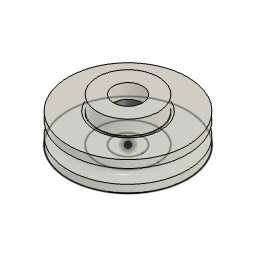
FilamentRoller v3 (Autodesk Fusion 360 design; units mm, degrees)
Autodesk Fusion 360 part; units mm, degrees
sketch "Main" plane through (0, 0, 0) normal (0, 0, 1) x (1, 0, 0)
  circle A0 centre (0, 0) radius 3.125
  circle A1 centre (0, 0) radius 6.125
  circle A2 centre (0, 0) radius 1.5
  dimension "d1" = 6.25
  dimension "d3" = 3
  dimension "d12" = 3
  constraint coincident A0.centre A1.centre
  measures "d1" diameter of A0
  measures "d12" diameter of A2
extrude "Extrude1" add sketch "Main" along normal blind 3 contours A1 makes body 1
sketch "Sketch2" plane through (0, 0, 0) normal (1, 0, 0) x (0, 1, 0)
  line L0 (6.125, 3) -> (-6.125, 3)
  line L1 (6.125, 0) -> (-6.125, 0)
  line L2 (6.125, 3) -> (6.125, 0)
  line L3 (6.125, 1.5) -> (5.125, 1.5) construction
  spline S0 degree 5 poles (6.125, 3) (6.125, 2.8466) (6.1777, 2.5757) (6.4146, 2.2769) (6.9886, 2.0773) (7.8292, 2.0694) (8.4441, 2.1927) (8.5459, 2.3381) (8.0488, 2.4223) (7.1302, 2.4004) (6.0916, 2.2496) (5.4387, 2.0191) (5.1775, 1.7838) (5.1226, 1.5992) (5.125, 1.5) knots 0 0 0 0 0 0 0.1 0.2 0.3 0.4 0.5 0.6 0.7 0.8 0.9 1 1 1 1 1 1
  line L4 (6.125, 3.25) -> (6.125, 2.75)
  line L5 (5.122, 1.6259) -> (5.128, 1.3741)
  spline S1 degree 5 poles (6.125, 0) (6.125, 0.1534) (6.1777, 0.4243) (6.4146, 0.7231) (6.9886, 0.9227) (7.8292, 0.9306) (8.4441, 0.8073) (8.5459, 0.6619) (8.0488, 0.5777) (7.1302, 0.5996) (6.0916, 0.7504) (5.4387, 0.9809) (5.1775, 1.2162) (5.1226, 1.4008) (5.125, 1.5) knots 0 0 0 0 0 0 0.1 0.2 0.3 0.4 0.5 0.6 0.7 0.8 0.9 1 1 1 1 1 1
  line L6 (6.125, -0.25) -> (6.125, 0.25)
  line L7 (5.122, 1.3741) -> (5.128, 1.6259)
  point P0 (8.4316, 2.2871)
  point P1 (8.4316, 0.7129)
  dimension "d8" = 1
  constraint coincident L0.start L2.start
  constraint coincident L1.start L2.end
  constraint midpoint L2 L3.start
  constraint perpendicular L2 L3
  constraint midpoint L0.start L4
  constraint coincident L2 L4.end
  constraint midpoint L3.end L5
  constraint symmetric S0.end L3 S1.end
  constraint symmetric L3 L0.start L1.start
  constraint symmetric L3 P0 P1
  constraint symmetric L3 L4.start L6.start
  constraint symmetric L3 L4.end L6.end
  constraint symmetric L3 L5.start L7.start
  constraint symmetric L3 L5.end L7.end
  measures "d8" distance of L3.start L3.end
revolve "Revolve1" cut sketch "Sketch2" angle 360 about axis through (0, 0, 0) along (0, 0, -1) contours L2 S0 S1 bodies 1
fillet "Fillet1" radius 0.25 2 edges at (-2.9135, 1.13, 3) (-2.9135, 1.13, 0) on bodies 1
extrude "Extrude2" add sketch "Main" along normal blind 3 separate body contours A0 makes body 2
sketch "Sketch3" plane through (0, 0, 3) normal (0, 0, 1) x (-1, 0, 0)
  circle A0 centre (0, 0) radius 1.5
  circle A1 centre (0, 0) radius 3.125
extrude "Extrude3" add sketch "Sketch3" along normal blind 1.5 separate body makes body 3
copy_body "CopyPasteBodies1" bodies 3 makes body 4
move_body "Move1" bodies 4 to x (1, 0, 0) y (0, 1, 0) z (0, 0, 1) at (0, 0, -4.5)
equation "d1 = bearingOD"
equation "bearingOD = 6.25 mm"
equation "bearingDepth = 3.0 mm"
equation "d5 = bearingDepth"
equation "d13 = bearingDepth"
named bodies: "FilamentRoller", "Bearing", "washer", "washer (1)"
